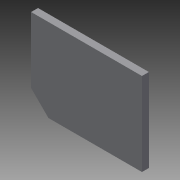
# Autodesk Inventor part: SD
Saved by Autodesk Inventor 2014 (Build 180170000, 170)
## iProperties
Created: 2013-05-24
Part Number: SD
Material: Generisch
Document SubType Name: Modeling
Designer: hartmann
Density: 1 g/cm^3
Appearance: Vorgabe
Author: hartmann
Autodesk Inventor part; units mm, degrees
ref_plane "YZ Plane" through (0, 0, 0) normal (1, 0, 0) x (0, 1, 0)
ref_plane "XZ Plane" through (0, 0, 0) normal (0, 1, 0) x (-1, 0, 0)
ref_plane "XY Plane" through (0, 0, 0) normal (0, 0, 1) x (1, 0, 0)
sketch "Skizze1" plane through (0, 0, 0) normal (0, 1, 0) x (-1, 0, 0)
  line L0 (0, 0) -> (32, 0)
  line L1 (32, 0) -> (32, 24)
  line L2 (32, 24) -> (0, 24)
  line L3 (0, 24) -> (0, 0)
  line L4 (32, 5) -> (27, 0)
  dimension "d0" = 32
  dimension "d1" = 24
  dimension "d2" = 45
  dimension "d3" = 19
  constraints: 10 end point, 2 parallel, 2 point on line, 1 horizontal, 1 perpendicular
  measures "d0" distance of L2.end L1.end
  measures "d1" distance of L0.end L1.end
  measures "d2" angle of L4 L1
  measures "d3" distance of L1.end L4.start
extrude "Extrusion1" add sketch "Skizze1" along normal blind 2 contours L3 L2 L1 L4 L0
